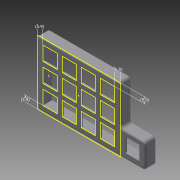
# Autodesk Inventor part: 13switch
Saved by Autodesk Inventor 2014 (Build 180170000, 170)
## iProperties
Created: 2016-02-13
Part Number: 13switch
Material: Generic
Document SubType Name: Modeling
Designer: Owner
Density: 1 g/cm^3
Appearance: Default
Author: Owner
Autodesk Inventor part; units mm, degrees
ref_plane "YZ Plane" through (0, 0, 0) normal (1, 0, 0) x (0, 1, 0)
ref_plane "XZ Plane" through (0, 0, 0) normal (0, 1, 0) x (-1, 0, 0)
ref_plane "XY Plane" through (0, 0, 0) normal (0, 0, 1) x (1, 0, 0)
sketch "Sketch1" plane through (0, 0, 0) normal (0, 1, 0) x (-1, 0, 0)
  line L0 (-41.6, -32.05) -> (41.6, -32.05)
  line L1 (41.6, -32.05) -> (41.6, 32.05)
  line L2 (41.6, 32.05) -> (-41.6, 32.05)
  line L3 (-41.6, 32.05) -> (-41.6, -32.05)
  line L4 (-41.6, -32.05) -> (41.6, 32.05) construction
  line L5 (41.6, -32.05) -> (-41.6, 32.05) construction
  point P0 (0, 0)
  dimension "d0" = 83.2
  dimension "d1" = 64.1
  constraints: 12 end point, 2 midpoint, 2 parallel, 1 horizontal, 1 perpendicular
  measures "d0" distance of L1.end L2.end
  measures "d1" distance of L0.end L1.end
extrude "Extrusion1" add sketch "Sketch1" along normal blind 10
sketch "Sketch2" plane through (0, 10, 0) normal (0, 1, 0) x (1, 0, 0)
  line L0 (41.6, 32.05) -> (-41.6, 32.05) projected
  line L1 (-41.6, 32.05) -> (-41.6, -32.05) projected
  line L2 (-36.6, 11.15) -> (-20.7, 11.15)
  line L3 (-20.7, 11.15) -> (-20.7, 27.05)
  line L4 (-20.7, 27.05) -> (-36.6, 27.05)
  line L5 (-36.6, 27.05) -> (-36.6, 11.15)
  line L6 (-36.6, 11.15) -> (-20.7, 27.05) construction
  line L7 (-20.7, 11.15) -> (-36.6, 27.05) construction
  point P0 (0, 0)
  point P1 (-28.65, 19.1)
  dimension "d4" = 5
  dimension "d5" = 5
  dimension "d6" = 15.9
  dimension "d7" = 15.9
  constraints: 12 end point, 2 midpoint, 2 parallel, 1 horizontal, 1 perpendicular
  measures "d4" distance between parallel lines of L1 L5
  measures "d5" distance between parallel lines of L0 L4
  measures "d6" distance of L3.end L4.end
  measures "d7" distance of L2.end L3.end
extrude "Extrusion2" cut sketch "Sketch2" against normal blind 8.4
sketch "Sketch3" plane through (0, 1.6, 0) normal (0, 1, 0) x (1, 0, 0)
  line L0 (-20.7, 27.05) -> (-20.7, 11.15) projected
  line L1 (-36.6, 27.05) -> (-20.7, 27.05) projected
  line L2 (-36.6, 27.05) -> (-20.7, 11.15) construction
  line L3 (-20.7, 27.05) -> (-36.6, 11.15) construction
  line L4 (-35.7, 12.05) -> (-21.6, 12.05)
  line L5 (-21.6, 12.05) -> (-21.6, 26.15)
  line L6 (-21.6, 26.15) -> (-35.7, 26.15)
  line L7 (-35.7, 26.15) -> (-35.7, 12.05)
  line L8 (-35.7, 12.05) -> (-21.6, 26.15) construction
  line L9 (-21.6, 12.05) -> (-35.7, 26.15) construction
  point P0 (0, 0)
  point P1 (-28.65, 19.1)
  dimension "d10" = 0.9
  dimension "d11" = 0.9
  constraints: 16 end point, 3 midpoint, 2 parallel, 2 perpendicular, 1 horizontal
  measures "d10" distance between parallel lines of L1 L6
  measures "d11" distance between parallel lines of L0 L5
extrude "Extrusion3" cut sketch "Sketch3" against normal through all
pattern_linear "Rectangular Pattern1" count 3 spacing 19.1 along (0, 0, 1) count 4 spacing 19.1 along (1, 0, 0) of "Extrusion2", "Extrusion3"
sketch "Sketch14" plane through (0, 0, 0) normal (0, -1, 0) x (1, 0, 0)
  line L0 (21.6, 12.05) -> (21.6, 26.15) projected
  line L1 (21.6, 26.15) -> (35.7, 26.15) projected
  line L2 (35.7, 26.15) -> (35.7, 12.05) projected
  line L3 (35.7, 12.05) -> (21.6, 12.05) projected
  line L4 (21.6, -7.05) -> (21.6, 7.05) projected
  line L5 (21.6, 7.05) -> (35.7, 7.05) projected
  line L6 (35.7, 7.05) -> (35.7, -7.05) projected
  line L7 (35.7, -7.05) -> (21.6, -7.05) projected
  line L8 (21.6, -26.15) -> (21.6, -12.05) projected
  line L9 (21.6, -12.05) -> (35.7, -12.05) projected
  line L10 (35.7, -12.05) -> (35.7, -26.15) projected
  line L11 (35.7, -26.15) -> (21.6, -26.15) projected
  line L12 (2.5, 12.05) -> (2.5, 26.15) projected
  line L13 (2.5, 26.15) -> (16.6, 26.15) projected
  line L14 (16.6, 26.15) -> (16.6, 12.05) projected
  line L15 (16.6, 12.05) -> (2.5, 12.05) projected
  line L16 (2.5, -7.05) -> (2.5, 7.05) projected
  line L17 (2.5, 7.05) -> (16.6, 7.05) projected
  line L18 (16.6, 7.05) -> (16.6, -7.05) projected
  line L19 (16.6, -7.05) -> (2.5, -7.05) projected
  line L20 (2.5, -26.15) -> (2.5, -12.05) projected
  line L21 (2.5, -12.05) -> (16.6, -12.05) projected
  line L22 (16.6, -12.05) -> (16.6, -26.15) projected
  line L23 (16.6, -26.15) -> (2.5, -26.15) projected
  line L24 (-16.6, 12.05) -> (-16.6, 26.15) projected
  line L25 (-16.6, 26.15) -> (-2.5, 26.15) projected
  line L26 (-2.5, 26.15) -> (-2.5, 12.05) projected
  line L27 (-2.5, 12.05) -> (-16.6, 12.05) projected
  line L28 (-16.6, -7.05) -> (-16.6, 7.05) projected
  line L29 (-16.6, 7.05) -> (-2.5, 7.05) projected
  line L30 (-2.5, 7.05) -> (-2.5, -7.05) projected
  line L31 (-2.5, -7.05) -> (-16.6, -7.05) projected
  line L32 (-16.6, -26.15) -> (-16.6, -12.05) projected
  line L33 (-16.6, -12.05) -> (-2.5, -12.05) projected
  line L34 (-2.5, -12.05) -> (-2.5, -26.15) projected
  line L35 (-2.5, -26.15) -> (-16.6, -26.15) projected
  line L36 (-35.7, 12.05) -> (-35.7, 26.15) projected
  line L37 (-35.7, 26.15) -> (-21.6, 26.15) projected
  line L38 (-21.6, 26.15) -> (-21.6, 12.05) projected
  line L39 (-21.6, 12.05) -> (-35.7, 12.05) projected
  line L40 (-35.7, -7.05) -> (-35.7, 7.05) projected
  line L41 (-35.7, 7.05) -> (-21.6, 7.05) projected
  line L42 (-21.6, 7.05) -> (-21.6, -7.05) projected
  line L43 (-21.6, -7.05) -> (-35.7, -7.05) projected
  line L44 (-21.6, -12.05) -> (-21.6, -26.15) projected
  line L45 (-21.6, -26.15) -> (-35.7, -26.15) projected
  line L46 (-35.7, -26.15) -> (-35.7, -12.05) projected
  line L47 (-35.7, -12.05) -> (-21.6, -12.05) projected
  line L48 (41.6, -32.05) -> (-41.6, -32.05) projected
  line L49 (41.6, 32.05) -> (41.6, -32.05) projected
  line L50 (-41.6, 32.05) -> (41.6, 32.05) projected
  line L51 (-41.6, -32.05) -> (-41.6, 32.05) projected
  point P0 (0, 0)
  dimension "d76" = 5.9
  dimension "d77" = 5.9
  dimension "d78" = 5.9
  dimension "d79" = 5.9
  measures "d76" distance between parallel lines of L51 L36
  measures "d77" distance between parallel lines of L49 L2
  measures "d78" distance between parallel lines of L48 L45
  measures "d79" distance between parallel lines of L50 L1
sketch "Sketch15" plane through (0, 0, 0) normal (0, -1, 0) x (1, 0, 0)
  line L0 (41.6, -32.05) -> (66.6, -32.05)
  line L1 (66.6, -32.05) -> (66.6, -7.05)
  line L2 (66.6, -7.05) -> (41.6, -7.05)
  line L3 (41.6, -7.05) -> (41.6, -32.05)
  point P0 (0, 0)
  dimension "d88" = 25
  dimension "d89" = 25
  constraints: 8 end point, 2 parallel, 1 horizontal, 1 perpendicular
  measures "d88" distance of L1.end L2.end
  measures "d89" distance of L0.end L1.end
extrude "Extrusion12" add sketch "Sketch15" against normal up to surface (10 mm away)
sketch "Sketch16" plane through (0, 0, 0) normal (0, -1, 0) x (1, 0, 0)
  line L0 (66.6, -32.05) -> (66.6, -7.05) projected
  line L1 (46.6, -12.05) -> (60.7, -12.05)
  line L2 (60.7, -12.05) -> (60.7, -26.15)
  line L3 (60.7, -26.15) -> (46.6, -26.15)
  line L4 (46.6, -26.15) -> (46.6, -12.05)
  point P0 (35.7, -12.05)
  point P1 (35.7, -26.15)
  point P2 (0, 0)
  dimension "d84" = 14.1
  dimension "d85" = 14.1
  dimension "d86" = 14.1
  dimension "d87" = 5.9
  constraints: 8 end point, 2 parallel, 1 horizontal, 1 perpendicular
  measures "d84" distance of point (35.7, -12.05) point (35.7, -26.15)
  measures "d85" distance of L3.end L1.start
  measures "d86" distance of L1.start L1.end
  measures "d87" distance between parallel lines of L0 L2
extrude "Extrusion13" cut sketch "Sketch16" against normal through all
sketch "Sketch17" plane through (0, 10, 0) normal (0, 1, 0) x (1, 0, 0)
  line L0 (46.6, 12.05) -> (46.6, 26.15) projected
  line L1 (46.6, 26.15) -> (60.7, 26.15) projected
  line L2 (60.7, 26.15) -> (60.7, 12.05) projected
  line L3 (60.7, 12.05) -> (46.6, 12.05) projected
  line L4 (36.6, 7.95) -> (36.6, -7.95) projected
  line L5 (61.6, 11.15) -> (61.6, 27.05)
  line L6 (61.6, 27.05) -> (45.7, 27.05)
  line L7 (45.7, 27.05) -> (45.7, 11.15)
  line L8 (45.7, 11.15) -> (61.6, 11.15)
  line L9 (35.7, -7.05) -> (35.7, 7.05) projected
  point P0 (0, 0)
  dimension "d92" = 0.9
  dimension "d93" = 0.9
  constraints: 8 end point, 3 other
  measures "d92" distance between parallel lines of L7 L0
  measures "d93" distance between parallel lines of L4 L9
extrude "Extrusion14" cut sketch "Sketch17" against normal up to surface (8.4 mm away)
fillet "Fillet4" radius 3 6 edges at (41.6, 5, 32.05) (41.6, 5, -7.05) (66.6, 5, -7.05) (66.6, 5, -32.05) (-41.6, 5, 32.05) (-41.6, 5, -32.05)
fillet "Fillet5" radius 2 12 edges at (40.7213, 0, 31.1713) (41.6, 0, 12.5) (42.4787, 0, -6.1713) (54.1, 0, -7.05) (65.7213, 0, -7.9287) (66.6, 0, -19.55) (65.7213, 0, -31.1713) (12.5, 0, -32.05) (-40.7213, 0, -31.1713) (-41.6, 0, 0) (-40.7213, 0, 31.1713) (0, 0, 32.05)
sketch "Sketch21" plane through (-41.6, 10, -29.05) normal (-1, 0, 0) x (0, 0, 1)
  line L0 (58.1, 0) -> (58.1, -8) projected
  line L1 (0, 0) -> (58.1, 0) projected
  line L2 (0, -8) -> (0, 0) projected
  line L3 (23.55, 0) -> (34.55, 0)
  line L4 (34.55, 0) -> (34.55, -4)
  line L5 (34.55, -4) -> (23.55, -4)
  line L6 (23.55, -4) -> (23.55, 0)
  line L7 (23.55, -2) -> (34.55, -2) construction
  line L8 (23.55, -2) -> (34.55, -2)
  line L9 (34.55, -2) -> (34.55, -4)
  line L10 (34.55, -4) -> (23.55, -4)
  line L11 (23.55, -4) -> (23.55, -2)
  point P0 (29.05, -10)
  dimension "d116" = 11
  dimension "d117" = 23.55
  dimension "d118" = 23.55
  dimension "d119" = 4
  constraints: 18 end point, 4 parallel, 2 horizontal, 2 midpoint, 2 perpendicular, 1 point on line
  measures "d116" distance of L3.start L3.end
  measures "d117" distance between parallel lines of L0 L4
  measures "d118" distance between parallel lines of L2 L6
  measures "d119" distance of L3.end L4.end
extrude "Extrusion18" cut sketch "Sketch21" against normal up to surface (78.2 mm away) contours L8 L4 L5 L6
sketch "Sketch22" plane through (36.6, 1.6, -7.95) normal (-1, 0, 0) x (0, 0, 1)
  line L0 (0, 8.4) -> (15.9, 8.4) projected
  line L1 (0, 8.4) -> (0, 0) projected
  line L2 (0, 0) -> (15.9, 0) projected
  line L3 (15.9, 8.4) -> (15.9, 0) projected
  line L4 (-24.1, 0.4) -> (-21.1, 0.4) projected
  line L5 (-24.1, 0.4) -> (-24.1, 8.4) projected
  line L6 (-24.1, 8.4) -> (-21.1, 8.4) projected
  line L7 (-21.1, 8.4) -> (-21.1, 0.4) projected
  line L8 (37, 0.4) -> (40, 0.4) projected
  line L9 (37, 0.4) -> (37, 8.4) projected
  line L10 (37, 8.4) -> (40, 8.4) projected
  line L11 (40, 8.4) -> (40, 0.4) projected
  line L12 (-21.1, 0.4) -> (-2.1, 0.4) projected
  line L13 (3.9, 0.4) -> (37, 0.4) projected
  line L14 (-2.1, 0.4) -> (0.9, 0.4) projected
  line L15 (3.9, 0.4) -> (0.9, 0.4) projected
  line L16 (-21.1, 8.4) -> (37, 8.4)
  line L17 (37, 8.4) -> (37, 0.4)
  line L18 (37, 0.4) -> (-21.1, 0.4)
  line L19 (-21.1, 0.4) -> (-21.1, 8.4)
  line L20 (-19.1, 8.4) -> (-19.1, 0) projected
  line L21 (35, 8.4) -> (35, 0) projected
  line L22 (-4.1, 0) -> (-18.2, 0) projected
  line L23 (15, 0) -> (0.9, 0) projected
  line L24 (-19.1, 8.4) -> (37, 8.4)
  line L25 (37, 8.4) -> (37, 0)
  line L26 (37, 0) -> (-19.1, 0)
  line L27 (-19.1, 0) -> (-19.1, 8.4)
  point P0 (7.95, -1.6)
  constraints: 16 end point, 4 parallel, 2 horizontal, 2 perpendicular
extrude "Extrusion19" cut sketch "Sketch22" along normal up to surface (73.2 mm away) contours L0 L3 L13 L15 L14 L1 | L1 L14 L12 L20 L16 | L16 L21 L13 L3 | L14 L15 L13 L3 L2 L1 | L1 L26 L22 L20 L12 L14 | L13 L21 L26 L3 | L16 L9 L13 L21 | L13 L25 L26 L21
sketch "Sketch23" plane through (36.6, 1.6, -27.05) normal (-1, 0, 0) x (0, 0, 1)
  line L0 (15.9, 0) -> (0, 0) projected
  line L1 (15.9, 8.4) -> (15.9, 0) projected
  line L2 (0, 8.4) -> (15.9, 8.4) projected
  line L3 (0, 8.4) -> (0, 0) projected
  point P0 (27.05, -1.6)
extrude "Extrusion20" cut sketch "Sketch23" against normal up to surface (25 mm away)
fillet "Fillet6" radius 3 1 edges at (36.6, 5.8, -11.15)
fillet "Fillet7" radius 1 2 edges at (-39.1, 8, -5.5) (-39.1, 8, 5.5)
equation "\"d5\" = d4"
equation "\"d7\" = d6"
equation "\"d11\" = d10"
body "Solid1"
